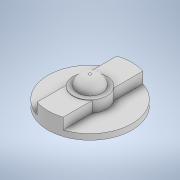
# Autodesk Inventor part: Деталь1
Saved by Autodesk Inventor 2020 (Build 240168000, 168)
## iProperties
Created: 2023-05-30
Part Number: Деталь1
Material: Типовые
Document SubType Name: Modeling
Designer: Qwellert
Density: 1 g/cm^3
Appearance: По умолчанию
Author: Qwellert
Autodesk Inventor part; units mm, degrees
ref_plane "YZ Plane" through (0, 0, 0) normal (1, 0, 0) x (0, 1, 0)
ref_plane "XZ Plane" through (0, 0, 0) normal (0, 1, 0) x (-1, 0, 0)
ref_plane "XY Plane" through (0, 0, 0) normal (0, 0, 1) x (1, 0, 0)
sketch "Эскиз1" plane through (0, 0, 0) normal (0, 1, 0) x (-1, 0, 0)
  circle A0 centre (0, 0) radius 9.815
  dimension "d0" = 19.63
  constraints: 1 centre point, 1 coincident
  measures "d0" diameter of A0
extrude "Выдавливание1" add sketch "Эскиз1" along normal blind 1.33
sketch "Эскиз2" plane through (0, 1.33, 0) normal (0, 1, 0) x (1, 0, 0)
  circle A0 centre (0, 0) radius 3.95
  dimension "d3" = 7.9
  constraints: 1 centre point, 1 coincident
  measures "d3" diameter of A0
extrude "Выдавливание2" add sketch "Эскиз2" along normal blind 2.7
sketch "Эскиз3" plane through (0, 4.03, 0) normal (0, 1, 0) x (1, 0, 0)
  circle A0 centre (0, 0) radius 2.845
  dimension "d6" = 5.69
  constraints: 1 centre point, 1 coincident
  measures "d6" diameter of A0
extrude "Выдавливание3" add sketch "Эскиз3" along normal blind 2.45
fillet "Сопряжение1" radius 2.5 1 edges at (-2.845, 6.48, 0)
sketch "Эскиз4" plane through (0, 1.33, 0) normal (0, 1, 0) x (1, 0, 0)
  circle A0 centre (0, 0) radius 9.815 projected
  line L0 (3.05, 9.815) -> (3.05, -9.815)
  line L1 (-3.05, 9.815) -> (-3.05, -9.815)
  point P0 (-3.05, 9.3291)
  point P1 (-3.05, -9.3291)
  point P2 (3.05, -9.3291)
  point P3 (3.05, 9.3291)
  constraints: 4 end point
extrude "Выдавливание4" add sketch "Эскиз4" along normal blind 2.6 contours L0 A0 L1
